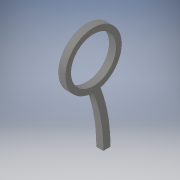
# Autodesk Inventor part: Mask holder2
Saved by Autodesk Inventor 2019.2 (Build 232265000, 265)
## iProperties
Created: 2020-09-20
Part Number: Mask holder2
Material: Generic
Document SubType Name: Modeling
Designer: SnoBotics
Density: 1 g/cm^3
Appearance: Rubber - Black(1)
Author: SnoBotics
Autodesk Inventor part; units mm, degrees
ref_plane "YZ Plane" through (0, 0, 0) normal (1, 0, 0) x (0, 1, 0)
ref_plane "XZ Plane" through (0, 0, 0) normal (0, 1, 0) x (-1, 0, 0)
ref_plane "XY Plane" through (0, 0, 0) normal (0, 0, 1) x (1, 0, 0)
sketch "Sketch1" plane through (0, 0, 0) normal (0, 0, 1) x (1, 0, 0)
  arc A0 (8.8174, -75.4289) -> (0, -25.4) centre (-130.8777, -74.2582) ccw
  line L0 (8.8174, -75.4289) -> (15.1687, -75.4289)
  arc A1 (15.1687, -75.4289) -> (6.2944, -24.6077) centre (-124.5198, -73.6357) ccw
  arc A2 (6.2944, -24.6077) -> (0, -25.4) centre (0, 0) ccw
  circle A3 centre (0, 0) radius 20.32
  point P0 (0, 0)
  dimension "d7" = 40.64
  constraints: 6 point on circle, 4 centre point, 2 end point, 1 coincident, 1 horizontal
  measures "d7" diameter of A3
extrude "Extrusion1" add sketch "Sketch1" along normal blind 6.35
sketch "Sketch2" plane through (0, 0, 6.35) normal (0, 0, 1) x (1, 0, 0)
  arc A0 (11.9924, -75.4289) -> (3.1501, -25.0035) centre (-127.6996, -73.9364) ccw construction
  line L0 (7.0984, -37.2544) -> (-17.2546, -44.4717)
  line L1 (-19.0349, -38.4646) -> (5.3181, -31.2472)
  arc A1 (7.0984, -37.2544) -> (5.3181, -31.2472) centre (6.2488, -34.2388) ccw
  line L2 (-42.5288, -26.9478) -> (-20.5002, -45.4336)
  line L3 (-20.5002, -45.4336) -> (-17.2546, -44.4717)
  line L4 (-38.4744, -22.1514) -> (-19.0349, -38.4646)
  line L5 (-40.3781, -18.0047) -> (-41.5692, -19.4938)
  line L6 (-45.5333, -19.4938) -> (-46.7244, -18.0047)
  arc A2 (-45.5333, -19.4938) -> (-41.5692, -19.4938) centre (-43.5513, -21.9717) ccw
  arc A3 (-46.7244, -18.0047) -> (-42.5288, -26.9478) centre (-43.5513, -21.9717) ccw
  arc A4 (-38.4744, -22.1514) -> (-40.3781, -18.0047) centre (-43.5513, -21.9717) ccw
  point P0 (0, 0)
  dimension "d13" = 50.4254
  constraints: 14 end point, 12 point on circle, 5 centre point, 2 concentric, 1 collinear, 1 parallel
  measures "d13" vertical distance of A0.start A0.end
sketch "Sketch3" plane through (0, 0, 0) normal (0, 0, -1) x (-1, 0, 0)
  arc A0 (-3.1501, -25.0035) -> (-11.9924, -75.4289) centre (127.6996, -73.9364) ccw construction
  line L0 (-7.0984, -37.2544) -> (17.2546, -44.4718)
  line L1 (19.0349, -38.4646) -> (-5.3181, -31.2472)
  arc A1 (-5.3181, -31.2472) -> (-7.0984, -37.2544) centre (-6.2487, -34.2388) ccw
  line L2 (42.5288, -26.9478) -> (20.5002, -45.4337)
  line L3 (20.5002, -45.4337) -> (17.2546, -44.4718)
  line L4 (38.4744, -22.1514) -> (19.0349, -38.4646)
  line L5 (40.3781, -18.0047) -> (41.5692, -19.4938)
  line L6 (45.5333, -19.4938) -> (46.7244, -18.0047)
  arc A2 (41.5692, -19.4938) -> (45.5333, -19.4938) centre (43.5513, -21.9717) ccw
  arc A3 (42.5288, -26.9478) -> (46.7244, -18.0047) centre (43.5513, -21.9717) ccw
  arc A4 (40.3781, -18.0047) -> (38.4744, -22.1514) centre (43.5513, -21.9717) ccw
  point P0 (0, 0)
  point P1 (0, 0)
  constraints: 14 end point, 12 point on circle, 5 centre point
body "Solid1"
